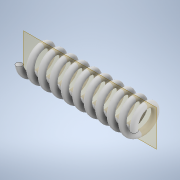
# Autodesk Inventor part: SecondaryCoil
Saved by Autodesk Inventor 2021 (Build 250183000, 183)
## iProperties
Created: 2022-02-09
Part Number: SecondaryCoil
Material: Generic
Document SubType Name: Modeling
Designer: tlar613
Density: 1 g/cm^3
Appearance: Default
Author: tlar613
Autodesk Inventor part; units mm, degrees
ref_plane "YZ Plane" through (0, 0, 0) normal (1, 0, 0) x (0, 1, 0)
ref_plane "XZ Plane" through (0, 0, 0) normal (0, 1, 0) x (-1, 0, 0)
sketch "Sketch3" plane through (0, 0, 0) normal (0, 1, 0) x (-1, 0, 0)
  circle A0 centre (0, 9.7) radius 2.15
  point P0 (0, 0)
  dimension "d2" = 4.3
  dimension "d3" = 9.7
  constraints: 1 centre point
  measures "d2" diameter of A0
  measures "d3" distance of point (0, 0) A0.centre
coil "Coil1" sketch "Sketch3" operation add axis through (-10, 0, 0) along (1, 0, 0) pitch 8.3 turns 10 hand right
body "Solid1"
